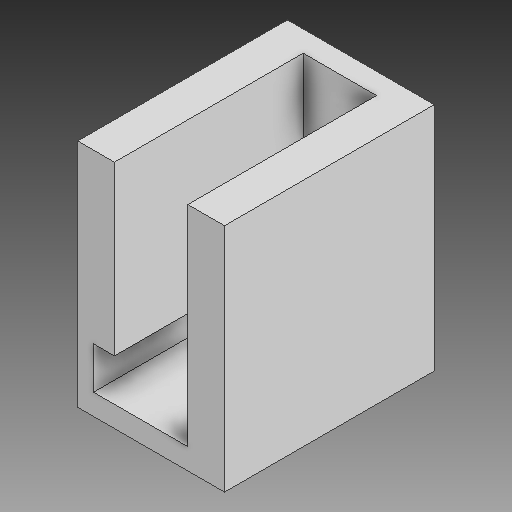
# Autodesk Inventor part: karmashek
Saved by Autodesk Inventor 2026 (Build 300175000, 175)
## iProperties
Created: 2025-11-12
Part Number: karmashek
Material: Типовые
Document SubType Name: Modeling
Designer: Admin
Density: 1 g/cm^3
Appearance: По умолчанию
Author: Admin
Autodesk Inventor part; units mm, degrees
ref_plane "YZ Plane" through (0, 0, 0) normal (1, 0, 0) x (0, 1, 0)
ref_plane "XZ Plane" through (0, 0, 0) normal (0, 1, 0) x (-1, 0, 0)
ref_plane "XY Plane" through (0, 0, 0) normal (0, 0, 1) x (1, 0, 0)
sketch "Эскиз1" plane through (0, 0, 0) normal (0, 0, 1) x (1, 0, 0)
  line L0 (7, -11) -> (-7, -11)
  line L1 (-7, -11) -> (-7, 11)
  line L2 (-7, 11) -> (7, 11)
  line L3 (7, 11) -> (7, -11)
  line L4 (7, -11) -> (-7, 11) construction
  line L5 (-7, -11) -> (7, 11) construction
  point P0 (0, 0)
  dimension "d0" = 14
  dimension "d1" = 22
  constraints: 12 end point, 2 midpoint, 2 parallel, 1 horizontal, 1 perpendicular
  measures "d0" distance of L1.end L2.end
  measures "d1" distance of L0.end L1.end
extrude "Выдавливание1" add sketch "Эскиз1" along normal blind 20
sketch "Эскиз2" plane through (0, 0, 20) normal (0, 0, 1) x (1, 0, 0)
  line L0 (7, 11) -> (-7, 11) projected
  line L1 (-3.5, 11) -> (3.5, 11)
  line L2 (3.5, 11) -> (3.5, -9)
  line L3 (3.5, -9) -> (-3.5, -9)
  line L4 (-3.5, -9) -> (-3.5, 11)
  point P0 (0, 0)
  dimension "d4" = 20
  dimension "d5" = 7
  dimension "d6" = 3.5
  constraints: 8 end point, 2 parallel, 1 horizontal, 1 perpendicular, 1 point on line
  measures "d4" distance of L3.end L1.start
  measures "d5" distance of L2.end L3.end
  measures "d6" distance from line of point (0, 0) L4
extrude "Выдавливание2" cut sketch "Эскиз2" against normal blind 18
sketch "Эскиз3" plane through (0, 0, 20) normal (0, 0, 1) x (1, 0, 0)
  line L0 (3.5, -9) -> (-3.5, -9) projected
  line L1 (-3.5, -9) -> (-5.5, -9)
  line L2 (-5.5, -9) -> (-5.5, -5)
  line L3 (-5.5, -5) -> (-3.5, -5)
  line L4 (-3.5, -5) -> (-3.5, -9)
  point P0 (0, 0)
  dimension "d9" = 2
  dimension "d10" = 4
  constraints: 8 end point, 2 parallel, 1 horizontal, 1 perpendicular
  measures "d9" distance of L0.end L1.end
  measures "d10" distance of L1.end L2.end
extrude "Выдавливание3" cut sketch "Эскиз3" against normal blind 20
